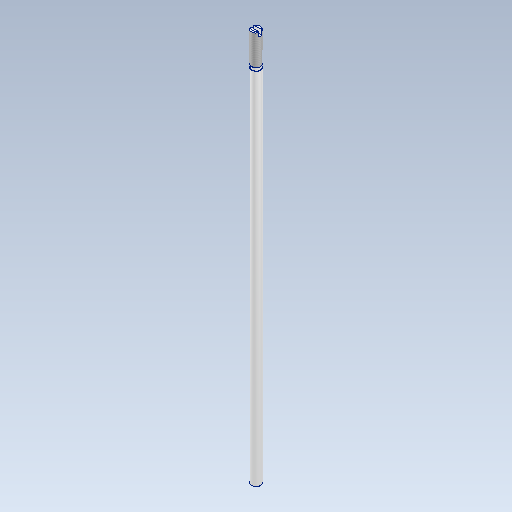
# Autodesk Inventor part: wał_prowadzący_hamulca_długi
Saved by Autodesk Inventor 2020 (Build 240168000, 168)
## iProperties
Created: 2020-08-31
Part Number: wał_prowadzący_hamulca_długi
Material: Aluminum 6061
Document SubType Name: Modeling
Designer: Hesekiel
Density: 2.7 g/cm^3
Appearance: Aluminum - Flat
Mass: 2.40755 g
Surface Area: 12.1432 cm^2
Volume: 0.891684 cm^3
Author: Hesekiel
Autodesk Inventor part; units mm, degrees
ref_plane "YZ Plane" through (0, 0, 0) normal (1, 0, 0) x (0, 1, 0)
ref_plane "XZ Plane" through (0, 0, 0) normal (0, 1, 0) x (-1, 0, 0)
ref_plane "XY Plane" through (0, 0, 0) normal (0, 0, 1) x (1, 0, 0)
sketch "Sketch1" plane through (0, 0, 0) normal (0, 1, 0) x (-1, 0, 0)
  circle A0 centre (0, 0) radius 1.5
  dimension "d0" = 3
  constraints: 1 centre point, 1 coincident
  measures "d0" diameter of A0
extrude "Extrusion1" add sketch "Sketch1" along normal blind 116
sketch "Sketch2" plane through (0, 116, 0) normal (0, 1, 0) x (1, 0, 0)
  circle A0 centre (0, 0) radius 1.4
  dimension "d3" = 2.8
  constraints: 1 centre point, 1 coincident
  measures "d3" diameter of A0
extrude "Extrusion2" add sketch "Sketch2" along normal blind 1
sketch "Sketch3" plane through (0, 117, 0) normal (0, 1, 0) x (1, 0, 0)
  circle A0 centre (0, 0) radius 1.5
  dimension "d6" = 3
  constraints: 1 centre point, 1 coincident
  measures "d6" diameter of A0
extrude "Extrusion3" add sketch "Sketch3" along normal blind 10
thread "Thread1" size "M3x0.5" class "6g" standard "ANSI Metric M Profile" full length
chamfer "Chamfer1" distance 0.3 angle 45 1 edges at (-1.5, 127, 0)
chamfer "Chamfer2" distance 0.3 angle 45 1 edges at (1.5, 0, 0)
sketch "Sketch4" plane through (0, 0, 0) normal (1, 0, 0) x (0, 1, 0)
  line L0 (117, -1.5) -> (117, 1.5) projected
  line L1 (126.7, -1.5) -> (126.7, 1.5) projected
  line L2 (126.7, -1.5) -> (126.7, 1.5) projected
  line L3 (127, 1.2) -> (127, -1.2) projected
  line L4 (128.5, 0.5) -> (125.5, 0.5)
  line L5 (125.5, 0.5) -> (125.5, -0.5)
  line L6 (125.5, -0.5) -> (128.5, -0.5)
  line L7 (128.5, -0.5) -> (128.5, 0.5)
  line L8 (127, 1.2) -> (127, -1.2) projected
  line L9 (128.5, 0.5) -> (125.5, -0.5) construction
  line L10 (125.5, 0.5) -> (128.5, -0.5) construction
  point P0 (0, 0)
  point P1 (127, 0)
  dimension "d17" = 3
  dimension "d18" = 1
  constraints: 12 end point, 3 midpoint, 2 parallel, 1 horizontal, 1 perpendicular
  measures "d17" distance of L6.end L5.end
  measures "d18" distance of L5.end L4.end
extrude "Extrusion4" cut sketch "Sketch4" along normal mid plane 10
body "Solid1"
